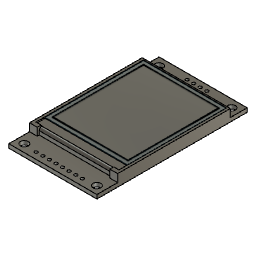
LCD_TFT_1.8_SPI_ST7735 v2 (Autodesk Fusion 360 design; units mm, degrees)
Autodesk Fusion 360 part; units mm, degrees
sketch "Sketch1" plane through (0, 0, 0) normal (0, 0, 1) x (1, 0, 0)
  line L0 (0, 0) -> (34, 0)
  line L1 (34, 0) -> (34, 58)
  line L2 (34, 58) -> (0, 58)
  line L3 (0, 58) -> (0, 0)
  circle A0 centre (3, 3) radius 1.5
  circle A1 centre (31, 3) radius 1.5
  circle A2 centre (3, 55) radius 1.5
  circle A3 centre (31, 55) radius 1.5
  dimension "d1" = 34
  dimension "d2" = 58
  dimension "d3" = 3
  dimension "d4" = 3
  dimension "d5" = 3
  dimension "d6" = 3
  dimension "d7" = 3
  dimension "d8" = 3
  dimension "d9" = 3
  dimension "d10" = 3
  dimension "d11" = 3
  dimension "d12" = 3
  dimension "d13" = 3
  dimension "d14" = 3
  constraint horizontal L0
  constraint vertical L1
  constraint horizontal L2
  constraint vertical L3
  constraint coincident L0.start L3.end
  measures "d1" distance of L0.start L0.end
  measures "d2" distance of L0.start L2.end
  measures "d3" diameter of A0
  measures "d4" distance of L3 A0.centre
  measures "d5" distance of L0 A0.centre
  measures "d6" diameter of A1
  measures "d7" distance of L1 A1.centre
  measures "d8" distance of L0 A1.centre
  measures "d9" diameter of A3
  measures "d10" diameter of A2
  measures "d11" distance of L2 A3.centre
  measures "d12" distance of L1 A3.centre
  measures "d13" distance of L2 A2.centre
  measures "d14" distance of L3 A2.centre
extrude "Extrude1" add sketch "Sketch1" along normal blind 1.5
sketch "Sketch2" plane through (0, 0, 1.5) normal (0, 0, 1) x (-1, 0, 0)
  circle A0 centre (-31, -3) radius 1.5
  circle A1 centre (-3, -55) radius 1.5
  circle A2 centre (-3, -3) radius 1.5
  circle A3 centre (-31, -55) radius 1.5
  line L0 (0, -58) -> (0, 0)
  line L1 (0, 0) -> (-34, 0)
  line L2 (-34, 0) -> (-34, -58)
  line L3 (-34, -58) -> (0, -58)
  line L4 (0, -8) -> (-34, -8)
  line L5 (-34, -8) -> (-34, -51.5)
  line L6 (-34, -51.5) -> (0, -51.5)
  line L7 (0, -51.5) -> (0, -8)
  dimension "d17" = 43.5
  dimension "d18" = 34
  dimension "d19" = 8
  constraint horizontal L4
  constraint vertical L5
  constraint horizontal L6
  constraint vertical L7
  constraint coincident L0 L4.start
  measures "d17" distance of L4.start L6.end
  measures "d18" distance of L5.end L6.end
  measures "d19" distance of L1 L4
extrude "Extrude2" add sketch "Sketch2" along normal blind 3 contours L0 L2 L4 L5 L6 L7
sketch "Sketch3" plane through (0, 0, 4.5) normal (0, 0, 1) x (-1, 0, 0)
  line L0 (0, -51.5) -> (0, -8)
  line L1 (0, -8) -> (-34, -8)
  line L2 (-34, -8) -> (-34, -51.5)
  line L3 (-34, -51.5) -> (0, -51.5)
  line L4 (-1, -13) -> (-33, -13)
  line L5 (-33, -13) -> (-33, -51)
  line L6 (-33, -51) -> (-1, -51)
  line L7 (-1, -51) -> (-1, -13)
  line L8 (-3, -13) -> (-31, -13)
  line L9 (-31, -13) -> (-31, -8)
  line L10 (-31, -8) -> (-3, -8)
  line L11 (-3, -8) -> (-3, -13)
  line L12 (-3, -9.5) -> (-1, -9.5)
  line L13 (-1, -9.5) -> (-1, -13)
  line L14 (-1, -13) -> (-3, -13)
  line L15 (-3, -13) -> (-3, -9.5)
  line L16 (-31, -9.5) -> (-33, -9.5)
  line L17 (-33, -9.5) -> (-33, -13)
  line L18 (-33, -13) -> (-31, -13)
  line L19 (-31, -13) -> (-31, -9.5)
  dimension "d22" = 5
  dimension "d23" = 0.5
  dimension "d24" = 1
  dimension "d25" = 1
  dimension "d38" = 28
  dimension "d39" = 3
  dimension "d42" = 1.5
  dimension "d43" = 1.5
  constraint perpendicular L4 L7
  constraint horizontal L8
  constraint vertical L9
  constraint horizontal L10
  constraint vertical L11
  constraint coincident L1 L9.end
  constraint coincident L4 L8.start
  constraint horizontal L12
  constraint vertical L13
  constraint horizontal L14
  constraint vertical L15
  constraint coincident L11 L12.start
  constraint horizontal L16
  constraint vertical L17
  constraint horizontal L18
  constraint vertical L19
  constraint coincident L9 L16.start
  measures "d22" distance of L1 L4
  measures "d23" distance of L3 L6
  measures "d24" distance of L2 L5
  measures "d25" distance of L0 L7
  measures "d38" distance of L9 L11
  measures "d39" distance of L0 L11
  measures "d42" distance of L1 L12
  measures "d43" distance of L1 L16
extrude "Extrude6" cut sketch "Sketch3" against normal blind 3 contours L4 L11 L12 L13 L14 L15 | L4 L9 L16 L17 L18 L19
extrude "Extrude5" cut sketch "Sketch3" against normal blind 3 contours L1 L4 L8 L9 L10 L11 L15 L19
sketch "Sketch4" plane through (0, 0, 1.5) normal (0, 0, 1) x (-1, 0, 0)
  line L0 (0, -58) -> (0, -51.5)
  line L1 (-34, -51.5) -> (-34, -58)
  circle A0 centre (-8.1, -2.5) radius 0.6
  circle A1 centre (-10.64, -2.5) radius 0.6
  circle A2 centre (-13.18, -2.5) radius 0.6
  circle A3 centre (-15.72, -2.5) radius 0.6
  circle A4 centre (-18.26, -2.5) radius 0.6
  circle A5 centre (-20.8, -2.5) radius 0.6
  circle A6 centre (-23.34, -2.5) radius 0.6
  circle A7 centre (-25.88, -2.5) radius 0.6
  line L2 (0, -51.5) -> (-34, -51.5)
  line L3 (-34, -58) -> (0, -58)
  circle A8 centre (-3, -55) radius 1.5
  circle A9 centre (-31, -55) radius 1.5
  dimension "d27" = 1.2
  dimension "d29" = 8.1
  dimension "d32" = -2.54
  dimension "d33" = 0
  measures "d27" diameter of A0
  measures "d29" distance of L0 A0.centre
extrude "Extrude3" cut sketch "Sketch4" against normal blind 1.5 contours A0 | A1 | A2 | A3 | A4 | A5 | A6 | A7
extrude "Extrude4" cut sketch "Sketch3" against normal blind 0.1 contours L4 L5 L6 L7 L8 L14 L18
extrude "Extrude7" cut sketch "Sketch3" against normal blind 0.2 contours L4 L5 L6 L7 L8 L14 L18
sketch "Sketch5" plane through (0, 0, 4.3) normal (0, 0, 1) x (-1, 0, 0)
  line L0 (-33, -51) -> (-1, -51)
  line L1 (-1, -51) -> (-1, -13)
  line L2 (-1, -13) -> (-33, -13)
  line L3 (-33, -13) -> (-33, -51)
  line L4 (-2.5, -49.5) -> (-31.5, -49.5)
  line L5 (-31.5, -49.5) -> (-31.5, -14.5)
  line L6 (-31.5, -14.5) -> (-2.5, -14.5)
  line L7 (-2.5, -14.5) -> (-2.5, -49.5)
  dimension "d48" = 1.5
  dimension "d49" = 1.5
  dimension "d50" = 1.5
  dimension "d51" = 1.5
  constraint horizontal L4
  constraint vertical L5
  constraint horizontal L6
  constraint vertical L7
  measures "d48" distance of L1 L7
  measures "d49" distance of L0 L4
  measures "d50" distance of L3 L5
  measures "d51" distance of L2 L6
extrude "Extrude8" add sketch "Sketch5" along normal blind 0.2 contours L4 L5 L6 L7
sketch "Sketch6" plane through (0, 0, 1.5) normal (0, 0, 1) x (-1, 0, 0)
  line L0 (0, -51.5) -> (-34, -51.5)
  line L1 (-34, -51.5) -> (-34, -58)
  line L2 (-34, -58) -> (0, -58)
  line L3 (0, -58) -> (0, -51.5)
  circle A0 centre (-3, -55) radius 1.5
  circle A1 centre (-31, -55) radius 1.5
  circle A2 centre (-13, -55.8) radius 0.6
  circle A3 centre (-15.54, -55.8) radius 0.6
  circle A4 centre (-18.08, -55.8) radius 0.6
  circle A5 centre (-20.62, -55.8) radius 0.6
  dimension "d54" = 1.2
  dimension "d55" = 13
  dimension "d56" = 2.2
  dimension "d59" = -2.54
  dimension "d60" = 0
  measures "d54" diameter of A2
  measures "d55" distance of L3 A2.centre
  measures "d56" distance of L2 A2.centre
extrude "Extrude9" cut sketch "Sketch6" against normal blind 1.5 contours A2 | A3 | A4 | A5
sketch "Sketch7" plane through (0, 0, 1.5) normal (0, 0, 1) x (-1, 0, 0)
  circle A0 centre (-20.8, -2.5) radius 0.6
  circle A1 centre (-10.64, -2.5) radius 0.6
  circle A2 centre (-13.18, -2.5) radius 0.6
  circle A3 centre (-23.34, -2.5) radius 0.6
  circle A4 centre (-18.26, -2.5) radius 0.6
  circle A5 centre (-8.1, -2.5) radius 0.6
  circle A6 centre (-15.72, -2.5) radius 0.6
  circle A7 centre (-25.88, -2.5) radius 0.6
  circle A8 centre (-3, -3) radius 1.5
  circle A9 centre (-31, -3) radius 1.5
  line L0 (-31, -9.5) -> (-33, -9.5)
  line L1 (-33, -9.5) -> (-33, -13)
  line L2 (-33, -13) -> (-1, -13)
  line L3 (-1, -13) -> (-1, -9.5)
  line L4 (-1, -9.5) -> (-3, -9.5)
  line L5 (-3, -9.5) -> (-3, -8)
  line L6 (-3, -8) -> (0, -8)
  line L7 (0, -8) -> (0, 0)
  line L8 (0, 0) -> (-34, 0)
  line L9 (-34, 0) -> (-34, -8)
  line L10 (-34, -8) -> (-31, -8)
  line L11 (-31, -8) -> (-31, -9.5)
  line L12 (-1, -13) -> (-33, -13)
  line L13 (-33, -13) -> (-33, -9.5)
  line L14 (-33, -9.5) -> (-1, -9.5)
  line L15 (-1, -9.5) -> (-1, -13)
  line L16 (-3, -9.5) -> (-31, -9.5)
  line L17 (-31, -9.5) -> (-31, -8.75)
  line L18 (-31, -8.75) -> (-3, -8.75)
  line L19 (-3, -8.75) -> (-3, -9.5)
  constraint horizontal L12
  constraint vertical L13
  constraint horizontal L14
  constraint vertical L15
  constraint coincident L0.end L1.start
  constraint coincident L2.end L3.start
  constraint horizontal L16
  constraint vertical L17
  constraint horizontal L18
  constraint vertical L19
  constraint midpoint L11 L17.end
  constraint coincident L4.end L5.start
extrude "Extrude10" add sketch "Sketch7" along normal blind 2.5 contours L0 L1 L2 L3 L4 L12 L13 L14 L15 L16 | L5 L11 L14 L16 L17 L18 L19
fillet "Fillet2" radius 1 1 edges at (17, 8.75, 4)
sketch "Sketch8" plane through (0, 0, 0) normal (0, 0, -1) x (1, 0, 0)
  circle A0 centre (15.54, -55.8) radius 0.6
  circle A1 centre (18.08, -55.8) radius 0.6
  circle A2 centre (13, -55.8) radius 0.6
  circle A3 centre (20.62, -55.8) radius 0.6
  circle A4 centre (20.8, -2.5) radius 0.6
  circle A5 centre (10.64, -2.5) radius 0.6
  circle A6 centre (13.18, -2.5) radius 0.6
  circle A7 centre (23.34, -2.5) radius 0.6
  circle A8 centre (18.26, -2.5) radius 0.6
  circle A9 centre (8.1, -2.5) radius 0.6
  circle A10 centre (15.72, -2.5) radius 0.6
  circle A11 centre (25.88, -2.5) radius 0.6
  circle A12 centre (31, -3) radius 1.5
  circle A13 centre (3, -55) radius 1.5
  circle A14 centre (3, -3) radius 1.5
  circle A15 centre (31, -55) radius 1.5
  line L0 (0, 0) -> (0, -58)
  line L1 (0, -58) -> (34, -58)
  line L2 (34, -58) -> (34, 0)
  line L3 (34, 0) -> (0, 0)
  line L4 (0, -19) -> (17, -19)
  line L5 (10, -45.5) -> (0, -45.5)
  line L6 (0, -45.5) -> (0, -19)
  line L7 (10, -45.5) -> (12.1213, -43.3787)
  line L8 (12.1213, -43.3787) -> (17, -43.3787)
  line L9 (17, -43.3787) -> (17, -19)
  dimension "d66" = 19
  dimension "d68" = 26.5
  dimension "d69" = 10
  dimension "d70" = 3
  dimension "d71" = 135
  constraint horizontal L4
  constraint horizontal L5
  constraint vertical L6
  constraint coincident L0 L4.start
  constraint parallel L4 L8
  constraint perpendicular L4 L9
  measures "d66" distance of L3 L4
  measures "d68" distance of L4 L5
  measures "d69" distance of L5.start L6
  measures "d70" distance of L5.start L7.end
  measures "d71" angle of L5 L7
extrude "Extrude11" add sketch "Sketch8" along normal blind 3 contours L0 L4 L5 L6 L7 L8 L9
sketch "Sketch9" plane through (0, 0, 0) normal (-1, 0, 0) x (0, -1, 0)
  line L0 (-58, 0) -> (-45.5, 0)
  line L1 (-45.5, 0) -> (-45.5, -3)
  line L2 (-45.5, -3) -> (-19, -3)
  line L3 (-19, -3) -> (-19, 0)
  line L4 (-19, 0) -> (0, 0)
  line L5 (0, 0) -> (0, 1.5)
  line L6 (0, 1.5) -> (-8, 1.5)
  line L7 (-8, 1.5) -> (-8, 4.5)
  line L8 (-8, 4.5) -> (-51.5, 4.5)
  line L9 (-51.5, 4.5) -> (-51.5, 1.5)
  line L10 (-51.5, 1.5) -> (-58, 1.5)
  line L11 (-58, 1.5) -> (-58, 0)
  line L12 (-45, -0.5) -> (-19.5, -0.5)
  line L13 (-19.5, -0.5) -> (-19.5, -2.5)
  line L14 (-19.5, -2.5) -> (-45, -2.5)
  line L15 (-45, -2.5) -> (-45, -0.5)
  dimension "d74" = 0.5
  dimension "d75" = 0.5
  dimension "d76" = 0.5
  dimension "d77" = 0.5
  constraint horizontal L12
  constraint vertical L13
  constraint horizontal L14
  constraint vertical L15
  measures "d74" distance of L2 L14
  measures "d75" distance of L1 L15
  measures "d76" distance of L3 L13
  measures "d77" distance of L4 L12
extrude "Extrude12" cut sketch "Sketch9" against normal blind 12.5 contours L12 L13 L14 L15
fillet "Fillet3" radius 0.3 8 edges at (5, 45.5, -3) (11.0607, 44.4393, -3) (14.5607, 43.3787, -3) (17, 31.1893, -3) (8.5, 19, -3) (17, 43.3787, -1.5) (10, 45.5, -1.5) (17, 19, -1.5)
sketch "Sketch10" plane through (0, 0, 0) normal (-1, 0, 0) x (0, -1, 0)
  arc A0 (-19.3, -3) -> (-19, -2.7) centre (-19.3, -2.7) ccw
  line L0 (-19, -2.7) -> (-19, 0)
  line L1 (-19, 0) -> (0, 0)
  line L2 (0, 0) -> (0, 1.5)
  line L3 (0, 1.5) -> (-8, 1.5)
  line L4 (-8, 1.5) -> (-8, 4.5)
  line L5 (-8, 4.5) -> (-51.5, 4.5)
  line L6 (-51.5, 4.5) -> (-51.5, 1.5)
  line L7 (-51.5, 1.5) -> (-58, 1.5)
  line L8 (-58, 1.5) -> (-58, 0)
  line L9 (-58, 0) -> (-45.5, 0)
  line L10 (-45.5, 0) -> (-45.5, -2.7)
  arc A1 (-45.5, -2.7) -> (-45.2, -3) centre (-45.2, -2.7) ccw
  line L11 (-45.2, -3) -> (-19.3, -3)
  line L12 (-19.5, -0.5) -> (-19.5, -2.5)
  line L13 (-19.5, -2.5) -> (-45, -2.5)
  line L14 (-45, -2.5) -> (-45, -0.5)
  line L15 (-45, -0.5) -> (-19.5, -0.5)
  line L16 (-45.5, 0) -> (-19, 0)
  line L17 (-19, 0) -> (-19, -3)
  line L18 (-19, -3) -> (-45.5, -3)
  line L19 (-45.5, -3) -> (-45.5, 0)
  constraint horizontal L16
  constraint vertical L17
  constraint horizontal L18
  constraint vertical L19
  constraint coincident L9.end L10.start
extrude "Extrude13" cut sketch "Sketch10" against normal blind 0.2 contours A0 L0 L10 A1 L11 L16 L17 L18 L19
